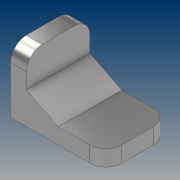
# Autodesk Inventor part: 33
Saved by Autodesk Inventor 2020.2 (Build 242310000, 310)
## iProperties
Created: 2020-09-17
Part Number: 33
Material: 鋼、碳鋼
Document SubType Name: Modeling
Designer: user
Density: 7.85 g/cm^3
Appearance: 半拋光
Mass: 307.262 g
Surface Area: 93.5106 cm^2
Volume: 39.1416 cm^3
Author: user
Autodesk Inventor part; units mm, degrees
ref_plane "YZ Plane" through (0, 0, 0) normal (1, 0, 0) x (0, 1, 0)
ref_plane "XZ Plane" through (0, 0, 0) normal (0, 1, 0) x (-1, 0, 0)
ref_plane "XY Plane" through (0, 0, 0) normal (0, 0, 1) x (1, 0, 0)
sketch "草圖1" plane through (0, 0, 0) normal (0, 1, 0) x (-1, 0, 0)
  line L0 (0, -20) -> (-60, -20)
  line L1 (-60, -20) -> (-60, 20)
  line L2 (-60, 20) -> (0, 20)
  line L3 (0, 20) -> (0, -20)
  point P0 (0, 0)
  point P1 (0, 0)
  dimension "d0" = 40
  dimension "d1" = 60
  constraints: 8 end point, 2 parallel, 1 coincident, 1 horizontal, 1 midpoint, 1 perpendicular
  measures "d0" distance of L2.end L0.start
  measures "d1" distance of L0.start L0.end
extrude "擠出1" add sketch "草圖1" along normal blind 40
sketch "草圖2" plane through (0, 0, 20) normal (0, 0, 1) x (1, 0, 0)
  line L0 (0, 0) -> (0, 40) projected
  line L1 (0, 40) -> (60, 40) projected
  line L2 (60, 40) -> (60, 0) projected
  line L3 (60, 0) -> (0, 0) projected
  line L4 (10, 40) -> (10, 20)
  line L5 (10, 20) -> (30, 10)
  line L6 (30, 10) -> (60, 10)
  line L7 (60, 0) -> (60, 40) projected
  dimension "d4" = 10
  dimension "d5" = 10
  dimension "d6" = 20
  dimension "d7" = 30
  constraints: 6 end point, 2 perpendicular, 2 point on line
  measures "d4" distance between parallel lines of L3 L6
  measures "d5" distance between parallel lines of L0 L4
  measures "d6" distance of L4.start L4.end
  measures "d7" distance of L5.end L6.end
extrude "擠出2" cut sketch "草圖2" against normal through all contours L1 L2 L6 L5 L4
fillet "圓角1" radius 10 4 edges at (5, 40, 20) (5, 40, -20) (60, 5, 20) (60, 5, -20)
